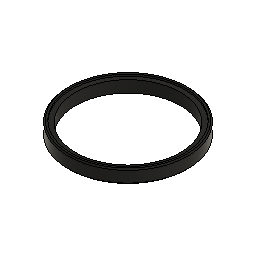
Parametric Exhaust Pipe (by FatalBulletHit) (Autodesk Fusion 360 design; units mm, degrees)
Autodesk Fusion 360 part; units mm, degrees
sketch "Sketch1" plane through (0, 0, 0) normal (1, 0, 0) x (0, 1, 0) in component "Parametric_ExhaustPipe_DOPM"
  line L0 (0, 0) -> (0, 4.4)
  line L1 (0, 0) -> (17.2, 0) construction
  line L2 (0, 0) -> (19.65, 0) construction
  line L3 (17.2, 0) -> (17.2, 3.8)
  line L4 (17.2, 3.8) -> (18.65, 3.8)
  line L5 (18.65, 3.8) -> (18.65, 4.4)
  line L6 (18.65, 4.4) -> (19.25, 4.4)
  line L7 (19.65, 4) -> (19.65, 0.4)
  line L8 (19.25, 0) -> (17.2, 0)
  line L9 (19.25, 4.4) -> (19.65, 4)
  line L10 (19.25, 0) -> (19.65, 0.4)
  point P0 (19.65, 4.4)
  point P1 (19.65, 0)
  dimension "d6" = 4.4
  dimension "d7" = 17.2
  dimension "d8" = 19.65
  dimension "d9" = 3.8
  dimension "d11" = 1.45
  dimension "d12" = 0.6
  dimension "d13" = 1
  dimension "d14" = 4.4
  dimension "d15" = 2.45
  dimension "d18" = 0.4
  dimension "d19" = 0.4
  dimension "d20" = 0.4
  dimension "d21" = 0.4
  constraint coincident L0.start L1.start
  constraint vertical L0
  constraint horizontal L1
  constraint horizontal L2
  constraint perpendicular L2 L3
  constraint perpendicular L3 L4
  constraint perpendicular L4 L5
  constraint perpendicular L5 L6
  constraint perpendicular L2 L7
  constraint perpendicular L3 L8
  constraint coincident P0 L6
  constraint coincident P0 L7
  constraint coincident P1 L8
  constraint coincident P1 L7
  measures "d6" distance of L0.start L0.end
  measures "d7" distance of L0.start L1.end
  measures "d8" distance of L0.start P1
  measures "d9" distance of L1.end L3.end
  measures "d11" distance of L3.end L4.end
  measures "d12" distance of L4.end L5.end
  measures "d13" distance of L5.end P0
  measures "d14" distance of P0 P1
  measures "d15" distance of P1 L1.end
  measures "d18" distance of P0 L6.end
  measures "d19" distance of P0 L7.start
  measures "d20" distance of P1 L8.start
  measures "d21" distance of P1 L7.end
revolve "Revolve1" add sketch "Sketch1" angle 360 about axis through (0, 0, 0) along (0, 0, 1) in component "Parametric_ExhaustPipe_DOPM"
component "Parametric_ExhaustPipe_DOPM" placed x (1, 0, 0) y (0, 1, 0) z (0, 0, 1) at (0, 0, 0)
equation "PanelThickness = 3 mm" comment "Default = 3.0"
equation "LipHeight = 0.6 mm" comment "Only adjust if needed // Max = 0.8 // Default = 0.6"
equation "ExcessHeight = 0.8 mm" comment "Only adjust if needed // Max = 1.0 // Default = 0.8"
equation "InnerDiameter = 34.4 mm" comment "Only adjust if needed // Default = 34.4"
equation "OuterDiameter = 39.3 mm" comment "Only adjust if needed // Default = 39.3"
equation "d6 = PanelThickness + LipHeight + ExcessHeight"
equation "d7 = InnerDiameter / 2"
equation "d8 = OuterDiameter / 2"
equation "d9 = PanelThickness + ExcessHeight"
equation "LipInnerDiameter = 37.3 mm" comment "Only adjust if needed // Default = 37.3"
equation "d11 = ( LipInnerDiameter - InnerDiameter ) / 2"
equation "d12 = LipHeight"
equation "d13 = ( OuterDiameter - LipInnerDiameter ) / 2"
equation "d14 = PanelThickness + LipHeight + ExcessHeight"
equation "d15 = ( OuterDiameter - InnerDiameter ) / 2"
equation "LipChamfer = 0.4 mm" comment "Only adjust if needed  // Default = 0.4"
equation "ExcessChamfer = 0.4 mm" comment "Only adjust if needed // Default = 0.4"
equation "d18 = LipChamfer"
equation "d19 = d18"
equation "d20 = ExcessChamfer"
equation "d21 = d20"
